Autodesk Inventor part; units mm, degrees
(part 4 of 4)
  arc A24 (22.4, -8.75) -> (27.75, -14.1) centre (27.75, -8.75) ccw
  line L1112 (27.75, -14.1) -> (37.6, -14.1)
  line L1113 (38.6, -14.1) -> (37.6, -14.1)
  line L1114 (16.1, -6.8) -> (16.4, -6.5)
  line L1115 (16.4, -6.5) -> (16.4, -6.35)
  line L1116 (15, -6.8) -> (16.1, -6.8)
  line L1117 (15.5343, -6.8) -> (16.1, -6.2343)
  circle A25 centre (15.55, -8.2) radius 0.225
  line L1118 (15.2, -7.9) -> (15.2, -8.2)
  arc A26 (15.2, -8.2) -> (15.9, -8.2) centre (15.55, -8.2) ccw
  line L1119 (15.9, -8.2) -> (15.9, -7.9)
  line L1120 (15, -7.9) -> (16.1, -7.9)
  line L1121 (3.1, -11.15) -> (14.0843, -11.15)
  line L1122 (14.0843, -11.15) -> (16.85, -8.3843)
  line L1123 (16.85, -8.3843) -> (16.85, -6.65)
  line L1124 (16.85, -6.65) -> (16.6743, -6.65)
  line L1125 (16.6743, -6.65) -> (16.4, -6.9243)
  line L1126 (16.4, -6.9243) -> (16.4, -8.2)
  line L1127 (16.4, -8.2) -> (16.2, -8.2)
  arc A27 (14.9, -8.2) -> (16.2, -8.2) centre (15.55, -8.2) ccw
  line L1128 (14.9, -8.2) -> (14.7, -8.2)
  line L1129 (14.7, -8.2) -> (14.7, -6.5)
  line L1130 (14.7, -6.5) -> (15.4101, -6.5)
  line L1131 (15.4101, -6.5) -> (15.8, -6.1101)
  line L1132 (15.8, -6.1101) -> (15.8, -4.2)
  line L1133 (16.4, 5.15) -> (16.1, 5.15) construction
  line L1134 (16.25, 5.15) -> (23.75, -5.15) construction
  line L1135 (23.9, -5.15) -> (23.6, -5.15) construction
  line L1136 (16.1, -5.15) -> (16.1, -6.35)
  line L1137 (16.1, -6.2343) -> (16.1, -6.35)
  line L1138 (16.4, -6.35) -> (16.1, -6.35)
  line L1139 (16.1, -6.35) -> (16.4, -6.35)
  line L1140 (16.1, -6.8) -> (15.5343, -6.8)
  line L1141 (15.2, -7.9) -> (15.9, -7.9)
  line L1142 (16.1, -7.9) -> (15, -7.9)
  line L1143 (27.9, -4.8) -> (28.2, -4.8)
  arc A28 (28.2, -4.8) -> (28.2, -4.1) centre (28.2, -4.45) ccw
  line L1144 (27.9, -4.8) -> (27.9, -4.1)
  circle A29 centre (28.2, -4.45) radius 0.225
  line L1145 (28.2, -4.1) -> (27.9, -4.1)
  line L1146 (26.5, -3.6) -> (26.35, -3.6)
  line L1147 (26.35, -3.9) -> (26.35, -3.6)
  line L1148 (26.2343, -3.9) -> (26.35, -3.9)
  line L1149 (26.8, -3.9) -> (26.5, -3.6)
  line L1150 (26.8, -4.4657) -> (26.2343, -3.9)
  line L1151 (26.8, -3.9) -> (26.8, -4.4657)
  line L1152 (24.8, 7.9) -> (24.8, 8.2)
  arc A30 (24.8, 8.2) -> (24.1, 8.2) centre (24.45, 8.2) ccw
  line L1153 (24.8, 7.9) -> (24.1, 7.9)
  circle A31 centre (24.45, 8.2) radius 0.225
  line L1154 (24.1, 8.2) -> (24.1, 7.9)
  line L1155 (23.6, 6.5) -> (23.6, 6.35)
  line L1156 (23.9, 6.35) -> (23.6, 6.35)
  line L1157 (23.9, 6.2343) -> (23.9, 6.35)
  line L1158 (23.9, 6.8) -> (23.6, 6.5)
  line L1159 (24.4657, 6.8) -> (23.9, 6.2343)
  line L1160 (23.9, 6.8) -> (24.4657, 6.8)
  line L1161 (12.1, 4.8) -> (11.8, 4.8)
  arc A32 (11.8, 4.8) -> (11.8, 4.1) centre (11.8, 4.45) ccw
  line L1162 (12.1, 4.8) -> (12.1, 4.1)
  circle A33 centre (11.8, 4.45) radius 0.225
  line L1163 (11.8, 4.1) -> (12.1, 4.1)
  line L1164 (13.5, 3.6) -> (13.65, 3.6)
  line L1165 (13.65, 3.9) -> (13.65, 3.6)
  line L1166 (13.7657, 3.9) -> (13.65, 3.9)
  line L1167 (13.2, 3.9) -> (13.5, 3.6)
  line L1168 (13.2, 4.4657) -> (13.7657, 3.9)
  line L1169 (13.2, 3.9) -> (13.2, 4.4657)
  line L1170 (15.8, -4.2) -> (13.35, -4.2)
  line L1171 (13.35, -4.2) -> (13.35, 3.3257)
  line L1172 (15.05, 10.05) -> (15.05, 9.75)
  line L1173 (15.75, 10.05) -> (14.65, 10.05)
  line L1174 (15.35, 10.05) -> (15.35, 9.75)
  line L1175 (16.1, 6.35) -> (16.1, 8.4)
  line L1176 (15.9, 8.6) -> (14.5, 8.6)
  line L1177 (16.1, 8.4) -> (15.9, 8.6)
  line L1178 (16.4, 6.35) -> (16.4, 8.5243)
  line L1179 (16.4, 8.5243) -> (15.9, 9.0243)
  line L1180 (16.9, 6.35) -> (16.9, 5.15)
  line L1181 (17.5, 7) -> (18.9, 7)
  line L1182 (16.6, 6.35) -> (16.6, 8.1243)
  line L1183 (17.65, 10.05) -> (18.75, 10.05)
  line L1184 (18.05, 10.05) -> (18.05, 9.75)
  line L1185 (18.35, 10.05) -> (18.35, 9.75)
  line L1186 (15.05, 10.05) -> (15.35, 10.05)
  line L1187 (18.05, 10.05) -> (18.35, 10.05)
  line L1188 (14.65, 10.05) -> (15.75, 10.05)
  line L1189 (23.4, 6.35) -> (23.4, 10.3536)
  line L1190 (23.1, 6.35) -> (23.1, 10.3536)
  line L1191 (22.3831, 10.3536) -> (23.4831, 10.3536)
  line L1192 (26.35, 3.75) -> (27.35, 3.75) construction
  arc A34 (27.35, 3.75) -> (31.35, 7.75) centre (27.35, 7.75) ccw construction
  line L1193 (31.35, 7.75) -> (31.35, 10.75) construction
  arc A35 (35.85, 15.25) -> (31.35, 10.75) centre (35.85, 10.75) ccw construction
  line L1194 (35.85, 15.25) -> (40.6, 15.25) construction
  line L1195 (26.35, 3.25) -> (27.35, 3.25) construction
  arc A36 (27.35, 3.25) -> (31.85, 7.75) centre (27.35, 7.75) ccw construction
  line L1196 (31.85, 7.75) -> (31.85, 10.75) construction
  arc A37 (35.85, 14.75) -> (31.85, 10.75) centre (35.85, 10.75) ccw construction
  line L1197 (35.85, 14.75) -> (40.6, 14.75) construction
  line L1198 (13.35, 3.3257) -> (13.0757, 3.6)
  line L1199 (13.0757, 3.6) -> (11.8, 3.6)
  line L1200 (12.1, 3.9) -> (13.2, 3.9) construction
  line L1201 (11.8, 3.6) -> (11.8, 3.8)
  arc A38 (11.8, 5.1) -> (11.8, 3.8) centre (11.8, 4.45) ccw
  line L1202 (11.8, 5.1) -> (11.8, 5.3)
  line L1203 (11.8, 5.3) -> (13.5, 5.3)
  line L1204 (13.5, 5.3) -> (13.5, 4.5899)
  line L1205 (13.5, 4.5899) -> (13.8899, 4.2)
  line L1206 (13.8899, 4.2) -> (15.9, 4.2)
  line L1207 (15.9, 4.2) -> (15.9, 7)
  line L1208 (14.5, 8.15) -> (14.2, 8.45)
  line L1209 (14.2, 8.45) -> (14.2, 11.45)
  line L1210 (14.2, 11.45) -> (19.2, 11.45)
  line L1211 (19.2, 11.45) -> (19.2, 8.45)
  line L1212 (19.2, 8.45) -> (18.9, 8.15)
  line L1213 (16.9, 6.35) -> (16.9, 8)
  line L1214 (16.9, 8) -> (17.5, 8.6)
  line L1215 (16.6, 8.1243) -> (17.5, 9.0243)
  line L1216 (17.5, 9.75) -> (17.5, 8.6)
  line L1217 (17.5, 7) -> (17.5, 6.65)
  line L1218 (17.5, 6.65) -> (22.8, 6.65)
  line L1219 (22.8, 6.65) -> (22.8, 10.0536)
  line L1220 (22.8, 10.0536) -> (22.0831, 10.0536)
  line L1221 (22.0831, 10.0536) -> (22.0831, 11.7536)
  line L1222 (22.0831, 11.7536) -> (23.7831, 11.7536)
  line L1223 (23.7831, 11.7536) -> (23.7831, 8.85)
  line L1224 (23.7831, 8.85) -> (24.45, 8.85)
  arc A39 (25.1, 8.2) -> (24.45, 8.85) centre (24.45, 8.2) ccw
  line L1225 (25.1, 8.2) -> (25.3, 8.2)
  line L1226 (25.3, 8.2) -> (25.3, 6.5)
  line L1227 (25.3, 6.5) -> (24.5899, 6.5)
  line L1228 (24.5899, 6.5) -> (24.2, 6.1101)
  line L1229 (24.2, 6.1101) -> (24.2, 4.6)
  line L1230 (24.2, 4.6) -> (27.35, 4.6)
  line L1231 (35.85, 15) -> (40.6, 15) construction
  line L1232 (40.6, 15.375) -> (35.85, 15.375)
  arc A40 (35.85, 15.375) -> (31.225, 10.75) centre (35.85, 10.75) ccw
  line L1233 (31.225, 10.75) -> (31.225, 7.75)
  arc A41 (27.35, 3.875) -> (31.225, 7.75) centre (27.35, 7.75) ccw
  line L1234 (27.35, 3.875) -> (26.35, 3.875)
  line L1235 (40.6, 15.125) -> (35.85, 15.125)
  arc A42 (35.85, 15.125) -> (31.475, 10.75) centre (35.85, 10.75) ccw
  line L1236 (31.475, 10.75) -> (31.475, 7.75)
  arc A43 (27.35, 3.625) -> (31.475, 7.75) centre (27.35, 7.75) ccw
  line L1237 (27.35, 3.625) -> (26.35, 3.625)
  line L1238 (40.6, 14.875) -> (35.85, 14.875)
  arc A44 (35.85, 14.875) -> (31.725, 10.75) centre (35.85, 10.75) ccw
  line L1239 (31.725, 10.75) -> (31.725, 7.75)
  arc A45 (27.35, 3.375) -> (31.725, 7.75) centre (27.35, 7.75) ccw
  line L1240 (27.35, 3.375) -> (26.35, 3.375)
  line L1241 (40.6, 14.625) -> (35.85, 14.625)
  arc A46 (35.85, 14.625) -> (31.975, 10.75) centre (35.85, 10.75) ccw
  line L1242 (31.975, 10.75) -> (31.975, 7.75)
  arc A47 (27.35, 3.125) -> (31.975, 7.75) centre (27.35, 7.75) ccw
  line L1243 (27.35, 3.125) -> (26.35, 3.125)
  line L1244 (26.35, 3.6) -> (26.35, 3.9)
  line L1245 (26.35, 3.1) -> (26.35, 3.4)
  line L1246 (40.6, 15.375) -> (40.6, 15.125)
  line L1247 (40.6, 14.875) -> (40.6, 14.625)
  arc A48 (27.35, 4.6) -> (30.5, 7.75) centre (27.35, 7.75) ccw
  line L1248 (30.5, 7.75) -> (30.5, 10.75)
  arc A49 (35.85, 16.1) -> (30.5, 10.75) centre (35.85, 10.75) ccw
  line L1249 (35.85, 16.1) -> (37.6, 16.1)
  line L1250 (37.6, 16.1) -> (38.6, 16.1)
  line L1251 (38.6, 16.1) -> (41.1, 16.1)
  line L1252 (41.1, 16.1) -> (41.1, 13.9)
  line L1253 (41.1, 13.9) -> (38.6, 13.9)
  line L1254 (38.6, -8.1) -> (38.6, -11.9)
  line L1255 (38.6, -11.9) -> (41.1, -11.9)
  line L1256 (41.1, -11.9) -> (41.1, -14.1)
  line L1257 (37.6, -14.1) -> (38.6, -14.1)
  line L1258 (41.1, -14.1) -> (38.6, -14.1)
  line L1259 (37.6, 13.9) -> (35.85, 13.9)
  arc A50 (35.85, 13.9) -> (32.7, 10.75) centre (35.85, 10.75) ccw
  line L1260 (32.7, 10.75) -> (32.7, 7.75)
  arc A51 (27.35, 2.4) -> (32.7, 7.75) centre (27.35, 7.75) ccw
  line L1261 (27.35, 2.4) -> (26.65, 2.4)
  line L1262 (26.65, 2.4) -> (26.65, -3.3257)
  line L1263 (26.65, -3.3257) -> (26.9243, -3.6)
  line L1264 (26.9243, -3.6) -> (28.2, -3.6)
  line L1265 (28.2, -3.6) -> (28.2, -3.8)
  arc A52 (28.2, -5.1) -> (28.2, -3.8) centre (28.2, -4.45) ccw
  line L1266 (28.2, -5.1) -> (28.2, -5.3)
  line L1267 (28.2, -5.3) -> (26.5, -5.3)
  line L1268 (26.5, -5.3) -> (26.5, -4.5899)
  line L1269 (26.5, -4.5899) -> (26.1101, -4.2)
  line L1270 (26.1101, -4.2) -> (24.6, -4.2)
  line L1271 (24.6, -4.2) -> (24.6, -8.75)
  arc A53 (24.6, -8.75) -> (27.75, -11.9) centre (27.75, -8.75) ccw
  line L1272 (37.6, -11.9) -> (37.6, -8.1)
  line L1273 (27.75, -11.9) -> (37.6, -11.9)
  circle A54 centre (18.5, -24.5) radius 0.175
  line L1274 (18.2, -25) -> (18.2, -24.5)
  arc A55 (18.8, -24.5) -> (18.2, -24.5) centre (18.5, -24.5) ccw
  line L1275 (18.8, -24.5) -> (18.8, -25)
  line L1276 (19, -25) -> (18, -25)
  line L1277 (18.2, -25) -> (18.8, -25)
  line L1278 (17.7, -27.8) -> (19.3, -27.8)
  line L1279 (19.3, -27.8) -> (19.3, -24.7)
  line L1280 (19.3, -24.7) -> (19.1, -24.7)
  line L1281 (19.1, -24.7) -> (19.1, -24.5)
  arc A56 (19.1, -24.5) -> (17.9, -24.5) centre (18.5, -24.5) ccw
  line L1282 (17.9, -24.5) -> (17.9, -24.7)
  line L1283 (17.9, -24.7) -> (17.7, -24.7)
  line L1284 (17.7, -24.7) -> (17.7, -27.8)
  line L1285 (18, -25) -> (18, -27.5)
  line L1286 (20.44, -24.7) -> (20.24, -24.7)
  line L1287 (21.84, -24.7) -> (21.64, -24.7)
  line L1288 (20.44, -24.5) -> (20.44, -24.7)
  line L1289 (21.64, -24.7) -> (21.64, -24.5)
  arc A57 (21.64, -24.5) -> (20.44, -24.5) centre (21.04, -24.5) ccw
  line L1290 (20.74, -25) -> (21.34, -25)
  line L1291 (21.34, -24.5) -> (21.34, -25)
  line L1292 (20.74, -25) -> (20.74, -24.5)
  arc A58 (21.34, -24.5) -> (20.74, -24.5) centre (21.04, -24.5) ccw
  circle A59 centre (21.04, -24.5) radius 0.175
  line L1293 (20.24, -24.7) -> (20.24, -27.8)
  line L1294 (20.24, -27.8) -> (21.84, -27.8)
  line L1295 (21.84, -27.8) -> (21.84, -24.7)
  line L1296 (22.98, -24.7) -> (22.78, -24.7)
  line L1297 (24.38, -24.7) -> (24.18, -24.7)
  line L1298 (22.98, -24.5) -> (22.98, -24.7)
  line L1299 (24.18, -24.7) -> (24.18, -24.5)
  arc A60 (24.18, -24.5) -> (22.98, -24.5) centre (23.58, -24.5) ccw
  line L1300 (23.28, -25) -> (23.88, -25)
  line L1301 (23.88, -24.5) -> (23.88, -25)
  line L1302 (23.28, -25) -> (23.28, -24.5)
  arc A61 (23.88, -24.5) -> (23.28, -24.5) centre (23.58, -24.5) ccw
  circle A62 centre (23.58, -24.5) radius 0.175
  line L1303 (22.78, -24.7) -> (22.78, -27.8)
  line L1304 (22.78, -27.8) -> (24.38, -27.8)
  line L1305 (24.38, -27.8) -> (24.38, -24.7)
  line L1306 (25.52, -24.7) -> (25.32, -24.7)
  line L1307 (26.92, -24.7) -> (26.72, -24.7)
  line L1308 (25.52, -24.5) -> (25.52, -24.7)
  line L1309 (26.72, -24.7) -> (26.72, -24.5)
  arc A63 (26.72, -24.5) -> (25.52, -24.5) centre (26.12, -24.5) ccw
  line L1310 (25.82, -25) -> (26.42, -25)
  line L1311 (26.42, -24.5) -> (26.42, -25)
  line L1312 (25.82, -25) -> (25.82, -24.5)
  arc A64 (26.42, -24.5) -> (25.82, -24.5) centre (26.12, -24.5) ccw
  circle A65 centre (26.12, -24.5) radius 0.175
  line L1313 (25.32, -24.7) -> (25.32, -27.8)
  line L1314 (25.32, -27.8) -> (26.92, -27.8)
  line L1315 (26.92, -27.8) -> (26.92, -24.7)
  line L1316 (28.06, -24.7) -> (27.86, -24.7)
  line L1317 (29.46, -24.7) -> (29.26, -24.7)
  line L1318 (28.06, -24.5) -> (28.06, -24.7)
  line L1319 (29.26, -24.7) -> (29.26, -24.5)
  arc A66 (29.26, -24.5) -> (28.06, -24.5) centre (28.66, -24.5) ccw
  line L1320 (28.36, -25) -> (28.96, -25)
  line L1321 (28.96, -24.5) -> (28.96, -25)
  line L1322 (28.36, -25) -> (28.36, -24.5)
  arc A67 (28.96, -24.5) -> (28.36, -24.5) centre (28.66, -24.5) ccw
  circle A68 centre (28.66, -24.5) radius 0.175
  line L1323 (27.86, -24.7) -> (27.86, -27.8)
  line L1324 (27.86, -27.8) -> (29.46, -27.8)
  line L1325 (29.46, -27.8) -> (29.46, -24.7)
  line L1326 (30.6, -24.7) -> (30.4, -24.7)
  line L1327 (32, -24.7) -> (31.8, -24.7)
  line L1328 (30.6, -24.5) -> (30.6, -24.7)
  line L1329 (31.8, -24.7) -> (31.8, -24.5)
  arc A69 (31.8, -24.5) -> (30.6, -24.5) centre (31.2, -24.5) ccw
  line L1330 (30.9, -25) -> (31.5, -25)
  line L1331 (31.5, -24.5) -> (31.5, -25)
  line L1332 (30.9, -25) -> (30.9, -24.5)
  arc A70 (31.5, -24.5) -> (30.9, -24.5) centre (31.2, -24.5) ccw
  circle A71 centre (31.2, -24.5) radius 0.175
  line L1333 (30.4, -24.7) -> (30.4, -27.8)
  line L1334 (30.4, -27.8) -> (32, -27.8)
  line L1335 (32, -27.8) -> (32, -24.7)
  point P0 (0, 0)
  point P1 (15.55, -7.9)
  point P2 (20, 0)
  point P3 (18.2, 10.05)
  point P4 (15.2, 10.05)
  point P5 (40.6, -12.75)
  point P6 (18.5, -25)
  point P7 (21.04, -25)
  point P8 (23.58, -25)
  point P9 (26.12, -25)
  point P10 (28.66, -25)
  point P11 (31.2, -25)
  dimension "d192" = 3
  dimension "d193" = 0.5
  dimension "d194" = 0.3
  dimension "d195" = 0.3
  dimension "d196" = 0.3
  dimension "d197" = 0.35
  dimension "d198" = 0.5
  dimension "d199" = 0.5
  dimension "d200" = 0.5
  dimension "d201" = 0.5
  dimension "d202" = 0.5
  dimension "d203" = 3
  dimension "d204" = 3
  dimension "d205" = 0.2
  dimension "d206" = 0.2
  dimension "d207" = 0.2
  dimension "d208" = 0.2
  dimension "d209" = 4
  dimension "d210" = 1.1
  dimension "d211" = 2
  dimension "d212" = 0.25
  dimension "d213" = 0.25
  dimension "d214" = 0.3
  dimension "d215" = 0.3
  dimension "d216" = 0.3
  dimension "d217" = 0.3
  dimension "d218" = 0.4
  dimension "d219" = 0.45
  dimension "d220" = 0.3
  dimension "d221" = 0.7
  dimension "d222" = 0.3
  dimension "d223" = 0.3
  dimension "d224" = 0.3
  dimension "d225" = 0.3
  dimension "d226" = 0.3
  dimension "d227" = 0.3
  dimension "d228" = 0.3
  dimension "d229" = 0.3
  dimension "d230" = 0.3
  dimension "d231" = 0.3
  dimension "d232" = 0.3
  dimension "d235" = 360
  dimension "d237" = 0.3
  dimension "d238" = 0.3
  dimension "d239" = 0.3
  dimension "d240" = 0.3
  dimension "d242" = 0.3
  dimension "d243" = 0.3
  dimension "d244" = 0.3
  dimension "d245" = 0.3
  dimension "d247" = 0.3
  dimension "d248" = 0.3
  dimension "d249" = 0.3
  dimension "d250" = 0.3
  dimension "d251" = 0.3
  dimension "d252" = 0.3
  dimension "d253" = 0.3
  dimension "d254" = 0.3
  dimension "d255" = 0.3
  dimension "d256" = 0.3
  dimension "d257" = 0.3
  dimension "d258" = 0.3
  dimension "d259" = 0.3
  dimension "d260" = 0.3
  constraints: 590 end point, 106 point on circle, 79 perpendicular, 75 point on line, 65 centre point, 39 tangent, 37 parallel, 30 concentric, 27 midpoint, 22 collinear, 21 horizontal, 15 vertical, 9 vertical alignment, 5 equal radius, 3 coincident, 303 other
  measures "d192" distance between parallel lines of L95 L996
  measures "d193" distance between parallel lines of L996 L1020
  measures "d194" distance between parallel lines of L989 L1022
  measures "d195" distance between parallel lines of L1037 L784
  measures "d196" distance between parallel lines of L1035 L1038
  measures "d197" diameter of A16
  measures "d198" distance of L1035.start L756.start
  measures "d199" distance of A12.centre A13.centre
  measures "d200" distance between parallel lines of L1047 L1044
  measures "d201" distance between parallel lines of L1050 L1047
  measures "d202" distance between parallel lines of L1054 L1050
  measures "d203" horizontal distance of L1043.end L1044.end
  measures "d204" horizontal distance of L1043.end L1044.end
  measures "d205" distance between parallel lines of L1061 L1058
  measures "d206" distance between parallel lines of L1067 L1064
  measures "d207" distance between parallel lines of L1073 L1070
  measures "d208" distance between parallel lines of L1079 L1076
  measures "d209" radius of A18
  measures "d210" distance between parallel lines of L1094 L163
  measures "d211" distance from line of L1091.end L162
  measures "d212" distance between parallel lines of L1099 L1101
  measures "d213" distance between parallel lines of L1095 L1097
  measures "d214" distance between parallel lines of L1107 L1081
  measures "d215" distance between parallel lines of L1108 L1080
  measures "d216" distance between parallel lines of L1109 L1079
  measures "d217" distance between parallel lines of L1110 L381
  measures "d218" distance between parallel lines of L1114 L1117
  measures "d219" diameter of A25
  measures "d220" distance from line of A25.centre L273
  measures "d221" distance between parallel lines of L1119 L1118
  measures "d222" distance between parallel lines of L1060 L1121
  measures "d223" distance between parallel lines of L1059 L1122
  measures "d224" distance between parallel lines of L1058 L1123
  measures "d225" distance between parallel lines of L1125 L1114
  measures "d226" distance between parallel lines of L1126 L272
  measures "d227" distance between parallel lines of L1127 L273
  measures "d228" radial gap between concentric circles of A27 A26
  measures "d229" distance between parallel lines of L1129 L274
  measures "d230" distance between parallel lines of L275 L1130
  measures "d231" distance between parallel lines of L1117 L1131
  measures "d232" distance between parallel lines of L406 L1132
  measures "d237" distance between parallel lines of L1170 L532
  measures "d238" distance between parallel lines of L533 L1171
  measures "d239" distance between parallel lines of L1174 L1172
  measures "d240" distance between parallel lines of L1179 L1177
  measures "d242" distance between parallel lines of L1185 L1184
  measures "d243" distance between parallel lines of L1214 L1215
  measures "d244" distance between parallel lines of L1198 L1167
  measures "d245" distance between parallel lines of L1199 L277
  measures "d247" distance between parallel lines of L279 L1203
  measures "d248" radial gap between concentric circles of A32 A38
  measures "d249" distance between parallel lines of L1168 L1205
  measures "d250" distance between parallel lines of L1204 L276
  measures "d251" distance between parallel lines of L343 L1206
  measures "d252" distance between parallel lines of L244 L1209
  measures "d253" distance between parallel lines of L554 L1210
  measures "d254" distance between parallel lines of L1211 L564
  measures "d255" distance between parallel lines of L427 L1218
  measures "d256" distance between parallel lines of L1190 L1219
  measures "d257" distance between parallel lines of L1220 L252
  measures "d258" distance between parallel lines of L1221 L253
  measures "d259" distance between parallel lines of L254 L1222
  measures "d260" distance between parallel lines of L1223 L255
extrude "Extrusion8" add sketch "Sketch8" along normal blind 0.05 contours L1249 A49 L1248 A48 L1230 L1229 L1228 L1227 L1226 L1225 A39 L1224 L1223 L1222 L1221 L1220 L1219 L1218 L1217 L251 L250 L1212 L1211 L1210 L1209 L1208 L568 L571 L1207 L1206 L1205 L1204 L1203 L1202 A38 L1201 L1199 L1198 L1171 L1170 L1132 L1131 L1130 L1129 L1128 A27 L1127 L1126 L1125 L1124 L1123 L1122 L1121 L1056 L1029 A9 L1030 L1041 L1040 A15 L1039 A14 L1038 L1037 L1032 A11 L1022 L1023 L1024 L1025 L1026 A7 L1027 L1057 L1107 L1108 L1109 L1110 L1111 A24 L1112 L180 L183 L182 L1258 L1256 L1255 L162 L161 L160 L1273 A53 L1271 L1270 L1269 L1268 L1267 L1266 A52 L1265 L1264 L1263 L1262 L1261 A51 L1260 A50 L1259 L48 L51 L50 L1253 L1252 L1251 L22 L21 L20 | L812 L1036 L756 L1035 A13 L1034 A12 L1033 | L644 L1078 L1077 L1076 L385 L1079 L1080 L1081 | L920 L1072 L1071 L1070 L389 L1073 L1074 L1075 | L648 L1066 L1065 L1064 L393 L1067 L1068 L1069 | L916 L1060 L1059 L1058 L397 L1061 L1062 L1063 | L997 L996 L995 L56 | L1002 L1001 L1000 L172 | L234 L1332 A70 L1331 | L238 L1312 A64 L1311 | L242 L1292 A58 L1291 | L246 L1179 L1178 L411 L1175 L1177 | L1172 L552 L1174 L245 | L1189 L467 L1190 L252 | L267 L1159 L468 L471 L1155 L1158 | L1154 A30 L1152 L265 | L271 L1150 L281 L280 L1146 L1149 | L1145 A28 L1143 L269 | L275 L1117 L406 L405 L1115 L1114 | L1119 A26 L1118 L273 | L1168 L343 L342 L1164 L1167 L276 | L278 L1163 A32 L1161 | L1240 A45 L1239 A44 L1238 L1247 L1241 A46 L1242 A47 L1243 L336 | L1095 A20 L1096 L1105 L1098 A21 L1097 L345 | L1099 A22 L1100 L1106 L1102 A23 L1101 L349 | L415 L1182 L1215 L566 L1214 L1213 | L1184 L556 L1185 L567 | L1234 A41 L1233 A40 L1232 L1246 L1235 A42 L1236 A43 L1237 L472 | L575 L1274 A55 L1275 | L578 L1302 A61 L1301 | L582 L1322 A67 L1321
equation "\"d23\" = d22"
equation "\"d25\" = d22"
equation "\"d12\" = d11"
equation "\"d91\" = d84"
equation "\"d96\" = d98"
body "Solid1"
